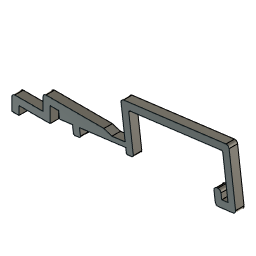
Hook arm over holder v17 (Autodesk Fusion 360 design; units mm, degrees)
Autodesk Fusion 360 part; units mm, degrees
note: some values were not read from the file. Set by a fixed rule: which sketch regions a step uses.
ref_plane "WorkPlane1" through (112.1576, 66, 17) normal (0, 1, 0) x (-1, 0, 0)
sketch "Sketch2" plane through (0, 66, 0) normal (0, 1, 0) x (1, 0, 0)
  line L0 (87, -6) -> (87, -28)
  line L1 (87, -28) -> (130, -28)
  line L2 (130, -28) -> (136, -26)
  line L3 (136, -26) -> (137, -23)
  line L4 (137, -23) -> (98, -18)
  line L5 (98, -18) -> (98, -23)
  line L6 (98, -23) -> (92, -23)
  line L7 (92, -23) -> (92, -6)
  line L8 (92, -6) -> (87, -6)
  constraint vertical L0
  constraint perpendicular L0 L1
  constraint perpendicular L1 L5
  constraint perpendicular L5 L6
  constraint perpendicular L6 L7
  constraint perpendicular L7 L8
extrude "Extrude1" add sketch "Sketch2" along normal blind 6 makes body 1
sketch "Sketch3" plane through (-0.6856, 0, 5.348) normal (0.127164, 0, -0.991882) x (0, 1, 0)
  line L0 (66, 138.8126) -> (66, 99.4934)
  line L1 (66, 99.4934) -> (72, 99.4934)
  line L2 (72, 99.4934) -> (72, 138.8126)
  line L3 (72, 138.8126) -> (66, 138.8126)
  line L4 (69.556, 99.4934) -> (69.556, 104.3824) construction
  line L5 (72, 104.3824) -> (66, 104.3824)
  line L6 (66, 104.3824) -> (66, 109.3824)
  line L7 (66, 109.3824) -> (72, 109.3824)
  line L8 (72, 109.3824) -> (72, 104.3824)
  line L9 (72, 109.3824) -> (66, 109.3824)
  line L10 (66, 109.3824) -> (66, 114.3824)
  line L11 (66, 114.3824) -> (72, 114.3824)
  line L12 (72, 114.3824) -> (72, 109.3824)
  dimension "d4" = 4.889
  dimension "d5" = 5
  dimension "d46" = 5
  constraint coincident L1 L4.start
  constraint perpendicular L1 L4
  constraint horizontal L5
  constraint vertical L6
  constraint horizontal L7
  constraint vertical L8
  constraint coincident L2 L5.start
  constraint horizontal L9
  constraint vertical L10
  constraint horizontal L11
  constraint vertical L12
  constraint coincident L0 L10.end
  measures "d4" distance of L4.start L4.end
  measures "d5" distance of L5.start L7.end
  measures "d46" distance of L7.end L11.end
sketch "Sketch4" plane through (0, 72, 0) normal (0, 1, 0) x (-1, 0, 0)
  line L0 (-137, 23) -> (-98, 18)
  line L1 (-98, 18) -> (-98, 23)
  line L2 (-98, 23) -> (-92, 23)
  line L3 (-92, 23) -> (-92, 6)
  line L4 (-92, 6) -> (-87, 6)
  line L5 (-87, 6) -> (-87, 28)
  line L6 (-87, 28) -> (-130, 28)
  line L7 (-130, 28) -> (-136, 26)
  line L8 (-136, 26) -> (-137, 23)
  line L9 (-87, 6) -> (-92, 6)
  line L10 (-92, 6) -> (-92, 12)
  line L11 (-92, 12) -> (-87, 12)
  line L12 (-87, 12) -> (-87, 6)
  line L13 (-87, 12) -> (-65, 12)
  line L14 (-65, 6) -> (-65, 12)
  line L15 (-65, 17) -> (-87, 17)
  line L16 (-65, 6) -> (-70, 6)
  line L17 (-70, 6) -> (-70, 12)
  line L18 (-70, 12) -> (-65, 12)
  line L19 (-65, 12) -> (-65, 6)
  line L20 (-65, 12) -> (-65, 17)
  constraint horizontal L9
  constraint vertical L10
  constraint horizontal L11
  constraint vertical L12
  constraint coincident L3 L10.end
  constraint coincident L4.end L5.start
  constraint perpendicular L5 L13
  constraint perpendicular L13 L14
  constraint midpoint L5 L15.end
  constraint perpendicular L5 L15
  constraint horizontal L16
  constraint vertical L17
  constraint horizontal L18
  constraint vertical L19
  constraint coincident L13 L17.end
  constraint perpendicular L18 L20
extrude "Extrude3" cut sketch "Sketch4" against normal blind 6.5 contours L3 L4 L5 L9 L10 L11 L12 bodies 1
extrude "Extrude4" add sketch "Sketch4" against normal blind 6 contours L5 L13 L15 L18 L20 | L13 L14 L16 L17 L18 L19 bodies 1
sketch "Sketch5" plane through (-0.6856, 0, 5.348) normal (0.127164, 0, -0.991882) x (0, 1, 0)
  line L0 (72, 99.4934) -> (72, 138.8126)
  line L1 (72, 138.8126) -> (66, 138.8126)
  line L2 (66, 138.8126) -> (66, 99.4934)
  line L3 (69, 109.3824) -> (69, 147.2714) construction
  line L4 (69, 147.2714) -> (66, 147.2714) construction
  line L5 (66, 147.2714) -> (66, 144.7714) construction
  line L6 (66, 144.7714) -> (69, 144.7714) construction
  line L7 (69, 144.7714) -> (69, 147.2714) construction
  line L8 (66, 144.7714) -> (72, 144.7714)
  line L9 (72, 144.7714) -> (72, 149.7714)
  line L10 (72, 149.7714) -> (66, 149.7714)
  line L11 (66, 149.7714) -> (66, 144.7714)
  line L12 (66, 99.4934) -> (72, 99.4934)
  dimension "d21" = 37.889
  dimension "d22" = 2.5
  dimension "d23" = 5
  constraint perpendicular L1 L3
  constraint horizontal L4
  constraint vertical L5
  constraint horizontal L6
  constraint vertical L7
  constraint horizontal L8
  constraint vertical L9
  constraint horizontal L10
  constraint vertical L11
  measures "d21" distance of L3.start L3.end
  measures "d22" distance of L3.end L6.end
  measures "d23" distance of L5.end L10.end
sketch "Sketch6" plane through (0, 66, 0) normal (0, -1, 0) x (1, 0, 0)
  line L0 (65, 17) -> (65, 6)
  line L1 (70, 12) -> (92, 12)
  line L2 (92, 12) -> (92, 23)
  line L3 (92, 23) -> (98, 23)
  line L4 (98, 23) -> (98, 18)
  line L5 (98, 18) -> (137, 23)
  line L6 (137, 23) -> (136, 26)
  line L7 (136, 26) -> (130, 28)
  line L8 (130, 28) -> (87, 28)
  line L9 (87, 28) -> (87, 17)
  line L10 (87, 17) -> (65, 17)
  line L11 (136.0676, 22.8805) -> (135.6529, 26.1157)
  line L12 (65, 6) -> (70, 6)
  line L13 (70, 6) -> (70, 12)
  constraint coincident L5 L11.start
  constraint coincident L7 L11.end
  constraint perpendicular L5 L11
extrude "Extrude5" cut sketch "Sketch6" against normal blind 6.8 contours L5 L6 L7 L11 bodies 1
extrude "Extrude6" add 1 faces at (135.9294, 68, 23.9589) along direction (0.991882, 0, 0.127164) blind 14.461 on bodies 1 bodies 1
sketch "Sketch7" plane through (-1.1004, 0, 8.5832) normal (-0.127164, 0, 0.991882) x (0, -1, 0)
  line L0 (-72, 137.8726) -> (-66, 137.8726)
  line L1 (-66, 137.8726) -> (-66, 152.3336)
  line L2 (-66, 152.3336) -> (-72, 152.3336)
  line L3 (-72, 152.3336) -> (-72, 137.8726)
  line L4 (-66, 152.3336) -> (-72.8279, 152.3336)
  line L5 (-72.8279, 152.3336) -> (-72.8279, 147.3336)
  line L6 (-72.8279, 147.3336) -> (-66, 147.3336)
  line L7 (-66, 147.3336) -> (-66, 152.3336)
  dimension "d30" = 5
  constraint horizontal L4
  constraint vertical L5
  constraint horizontal L6
  constraint vertical L7
  constraint coincident L1.end L2.start
  measures "d30" distance of L1.end L6.end
extrude "Extrude8" add sketch "Sketch7" along normal blind 30 contours L1 L2 L3 L4 L6 L7 bodies 1
sketch "Sketch8" plane through (151.0969, 0, 19.3714) normal (0.991882, 0, 0.127164) x (0, 1, 0)
  line L0 (72, 5.3918) -> (72, 38.6535)
  line L1 (72, 38.6535) -> (66, 38.6535)
  line L2 (66, 38.6535) -> (66, 5.3918)
  line L3 (66, 38.6535) -> (72, 38.6535)
  line L4 (72, 38.6535) -> (72, 33.6535)
  line L5 (72, 33.6535) -> (66, 33.6535)
  line L6 (66, 33.6535) -> (66, 38.6535)
  line L7 (66, 5.3918) -> (72, 5.3918)
  dimension "d33" = 5
  constraint horizontal L3
  constraint vertical L4
  constraint horizontal L5
  constraint vertical L6
  constraint coincident L1.end L2.start
  measures "d33" distance of L1.end L5.end
extrude "Extrude9" add sketch "Sketch8" along normal blind 72 contours L0 L1 L2 L3 L4 L5 L6 bodies 1
sketch "Sketch9" plane through (-4.2795, 0, 33.3803) normal (0.127164, 0, -0.991882) x (0, 1, 0)
  line L0 (66, 152.3336) -> (72, 152.3336)
  line L1 (72, 152.3336) -> (72, 224.3336)
  line L2 (72, 224.3336) -> (66, 224.3336)
  line L3 (66, 224.3336) -> (66, 152.3336)
  line L4 (72, 224.3336) -> (66, 224.3336)
  line L5 (66, 224.3336) -> (66, 219.3336)
  line L6 (66, 219.3336) -> (72, 219.3336)
  line L7 (72, 219.3336) -> (72, 224.3336)
  dimension "d36" = 5
  constraint horizontal L4
  constraint vertical L5
  constraint horizontal L6
  constraint vertical L7
  constraint coincident L3 L5.end
  constraint coincident L1.end L2.start
  measures "d36" distance of L1.end L6.end
extrude "Extrude10" add sketch "Sketch9" along normal blind 40 contours L1 L2 L3 L4 L5 L6 L7 bodies 1
sketch "Sketch10" plane through (0.807, 0, -6.295) normal (0.127164, 0, -0.991882) x (0, 1, 0)
  line L0 (72, 219.3336) -> (72, 224.3336)
  line L1 (72, 224.3336) -> (66, 224.3336)
  line L2 (66, 224.3336) -> (66, 219.3336)
  line L3 (66, 219.3336) -> (72, 219.3336)
  line L4 (66, 219.3336) -> (72.721, 219.3336)
  line L5 (66, 214.8336) -> (66, 219.3336)
  line L6 (72, 219.3336) -> (66, 219.3336)
  line L7 (66, 219.3336) -> (66, 214.8336)
  line L8 (66, 214.8336) -> (72, 214.8336)
  line L9 (72, 214.8336) -> (72, 219.3336)
  line L10 (66, 214.8336) -> (72, 214.8336)
  line L11 (72, 214.8336) -> (72, 209.8336)
  line L12 (72, 209.8336) -> (66, 209.8336)
  line L13 (66, 209.8336) -> (66, 214.8336)
  dimension "d40" = 6
  dimension "d41" = 4.5
  dimension "d56" = 5
  constraint horizontal L4
  constraint vertical L5
  constraint coincident L2.end L3.start
  constraint horizontal L6
  constraint vertical L7
  constraint horizontal L8
  constraint vertical L9
  constraint coincident L0.start L3.end
  constraint horizontal L10
  constraint vertical L11
  constraint horizontal L12
  constraint vertical L13
  measures "d40" distance of L0.start L2.end
  measures "d41" distance of L0.start L8.end
  measures "d56" distance of L5.start L12.end
extrude "Extrude11" add sketch "Sketch10" against normal blind 5 contours L3 L4 L5 L6 L7 L8 L9 L10 bodies 1
extrude "Extrude13" add sketch "Sketch3" along normal blind 6 contours L0 L2 L7 L9 L10 L11 L12 bodies 1
sketch "Sketch11" plane through (-0.6856, 0, 5.348) normal (0.127164, 0, -0.991882) x (0, 1, 0)
  line L0 (66, 114.3824) -> (72, 114.3824)
  line L1 (72, 114.3824) -> (72, 152.3336)
  line L2 (72, 152.3336) -> (66, 152.3336)
  line L3 (66, 152.3336) -> (66, 114.3824)
  line L4 (72, 152.3336) -> (65.9909, 152.3336)
  line L5 (65.9909, 152.3336) -> (65.9909, 147.3336)
  line L6 (65.9909, 147.3336) -> (72, 147.3336)
  line L7 (72, 147.3336) -> (72, 152.3336)
  dimension "d49" = 5
  constraint horizontal L4
  constraint vertical L5
  constraint horizontal L6
  constraint vertical L7
  constraint coincident L1.end L2.start
  measures "d49" distance of L1.end L6.end
extrude "Extrude14" add sketch "Sketch11" along normal blind 4 contours L1 L2 L3 L4 L6 L7 bodies 1
fillet "Fillet4" radius 1 2 edges at (113.5311, 69, 13.9421) (108.5717, 69, 13.3062) on bodies 1
fillet "Fillet5" radius 1 2 edges at (145.9605, 69, 20.116) (150.9199, 69, 20.7519) on bodies 1
extrude "Extrude15" add sketch "Sketch10" against normal blind 11 separate body contours L8 L10 L11 L12 L13 makes body 2
fillet "Fillet6" radius 2 4 edges at (223.3194, 69, 22.2322) (212.4977, 69, 31.9349) (207.5383, 69, 31.2991) (208.9371, 69, 20.3884) on bodies 1 2
sketch "Sketch12" plane through (0, 66, 0) normal (0, -1, 0) x (1, 0, 0)
  arc A0 (221.3356, 21.9779) -> (223.0651, 24.216) centre (221.0813, 23.9617) ccw
  line L0 (223.0651, 24.216) -> (217.597, 66.8669)
  line L1 (217.597, 66.8669) -> (141.2221, 57.0753)
  line L2 (141.2221, 57.0753) -> (145.037, 27.3188)
  line L3 (145.037, 27.3188) -> (135.6529, 26.1157)
  line L4 (135.6529, 26.1157) -> (130, 28)
  line L5 (130, 28) -> (87, 28)
  line L6 (87, 28) -> (87, 17)
  line L7 (87, 17) -> (65, 17)
  line L8 (65, 17) -> (65, 6)
  line L9 (65, 6) -> (70, 6)
  line L10 (70, 6) -> (70, 12)
  line L11 (70, 12) -> (92, 12)
  line L12 (92, 12) -> (92, 23)
  line L13 (92, 23) -> (98, 23)
  line L14 (98, 23) -> (98, 18)
  line L15 (98, 18) -> (107.8087, 19.2575)
  line L16 (107.8087, 19.2575) -> (108.4445, 14.2981)
  arc A1 (108.4445, 14.2981) -> (109.5636, 13.4334) centre (109.4364, 14.4253) ccw
  line L17 (109.5636, 13.4334) -> (112.5392, 13.8149)
  arc A2 (112.5392, 13.8149) -> (113.4039, 14.9339) centre (112.4121, 14.8068) ccw
  line L18 (113.4039, 14.9339) -> (112.7681, 19.8933)
  line L19 (112.7681, 19.8933) -> (145.4518, 24.0836)
  line L20 (145.4518, 24.0836) -> (145.8333, 21.1079)
  arc A3 (145.8333, 21.1079) -> (146.9524, 20.2432) centre (146.8252, 21.2351) ccw
  line L21 (146.9524, 20.2432) -> (149.928, 20.6247)
  arc A4 (149.928, 20.6247) -> (150.7927, 21.7437) centre (149.8008, 21.6166) ccw
  line L22 (150.7927, 21.7437) -> (146.8173, 52.7517)
  line L23 (146.8173, 52.7517) -> (213.2734, 61.2717)
  line L24 (213.2734, 61.2717) -> (217.7242, 26.5558)
  line L25 (217.7242, 26.5558) -> (213.2607, 25.9836)
  line L26 (213.2607, 25.9836) -> (213.8965, 21.0242)
  line L27 (213.8965, 21.0242) -> (221.3356, 21.9779)
  line L28 (98, 23) -> (98.6307, 18.0809)
  constraint coincident L13.end L14.start
  constraint coincident L15 L28.end
  constraint perpendicular L15 L28
extrude "Extrude16" cut sketch "Sketch12" against normal blind 8 contours L14 L15 L28 bodies 1
fillet "Fillet7" radius 2 2 edges at (87, 69, 28) (65, 69, 17) on bodies 1
fillet "Fillet8" radius 2 2 edges at (141.2221, 69, 57.0753) (217.597, 69, 66.8669) on bodies 1
fillet "Fillet8" radius 2.5 2 edges at (146.8173, 69, 52.7517) (213.2734, 69, 61.2717) on bodies 1
sketch "Sketch13" plane through (0, 66, 0) normal (0, -1, 0) x (1, 0, 0)
  arc A0 (217.8513, 64.8832) -> (215.6132, 66.6126) centre (215.8676, 64.6288) ccw
  line L0 (215.6132, 66.6126) -> (143.2059, 57.3296)
  arc A1 (143.2059, 57.3296) -> (141.4764, 55.0915) centre (143.4602, 55.3458) ccw
  line L1 (141.4764, 55.0915) -> (145.037, 27.3188)
  line L2 (145.037, 27.3188) -> (135.6529, 26.1157)
  line L3 (135.6529, 26.1157) -> (130, 28)
  line L4 (130, 28) -> (89, 28)
  arc A2 (89, 28) -> (87, 26) centre (89, 26) ccw
  line L5 (87, 26) -> (87, 17)
  line L6 (87, 17) -> (67, 17)
  arc A3 (67, 17) -> (65, 15) centre (67, 15) ccw
  line L7 (65, 15) -> (65, 6)
  line L8 (65, 6) -> (70, 6)
  line L9 (70, 6) -> (70, 12)
  line L10 (70, 12) -> (92, 12)
  line L11 (92, 12) -> (92, 23)
  line L12 (92, 23) -> (98, 23)
  line L13 (98, 23) -> (98.6307, 18.0809)
  line L14 (98.6307, 18.0809) -> (107.8087, 19.2575)
  line L15 (107.8087, 19.2575) -> (108.4445, 14.2981)
  arc A4 (108.4445, 14.2981) -> (109.5636, 13.4334) centre (109.4364, 14.4253) ccw
  line L16 (109.5636, 13.4334) -> (112.5392, 13.8149)
  arc A5 (112.5392, 13.8149) -> (113.4039, 14.9339) centre (112.4121, 14.8068) ccw
  line L17 (113.4039, 14.9339) -> (112.7681, 19.8933)
  line L18 (112.7681, 19.8933) -> (145.4518, 24.0836)
  line L19 (145.4518, 24.0836) -> (145.8333, 21.1079)
  arc A6 (145.8333, 21.1079) -> (146.9524, 20.2432) centre (146.8252, 21.2351) ccw
  line L20 (146.9524, 20.2432) -> (149.928, 20.6247)
  arc A7 (149.928, 20.6247) -> (150.7927, 21.7437) centre (149.8008, 21.6166) ccw
  line L21 (150.7927, 21.7437) -> (147.1353, 50.272)
  arc A8 (149.2971, 53.0696) -> (147.1353, 50.272) centre (149.615, 50.5899) ccw
  line L22 (149.2971, 53.0696) -> (210.7937, 60.9538)
  arc A9 (213.5913, 58.792) -> (210.7937, 60.9538) centre (211.1116, 58.4741) ccw
  line L23 (213.5913, 58.792) -> (217.7242, 26.5558)
  line L24 (217.7242, 26.5558) -> (213.2607, 25.9836)
  line L25 (213.2607, 25.9836) -> (213.8965, 21.0242)
  line L26 (213.8965, 21.0242) -> (221.3356, 21.9779)
  arc A10 (221.3356, 21.9779) -> (223.0651, 24.216) centre (221.0813, 23.9617) ccw
  line L27 (223.0651, 24.216) -> (217.8513, 64.8832)
  line L28 (180.0454, 57.0117) -> (180.6812, 52.0523)
  line L29 (180.6812, 52.0523) -> (213.9092, 56.3123)
  line L30 (180.6812, 52.0523) -> (147.4532, 47.7923)
  dimension "d69" = 5
  constraint midpoint L22 L28.start
  constraint perpendicular L22 L28
  constraint coincident L23 L29.end
  constraint perpendicular L23 L29
  constraint coincident L21 L30.end
  constraint perpendicular L21 L30
  measures "d69" distance of L28.start L28.end
extrude "Extrude17" add sketch "Sketch13" against normal blind 6 contours L22 A9 L23 L28 L29 | L21 A8 L22 L28 L30 bodies 1
sketch "Sketch14" plane through (0, 66, 0) normal (0, -1, 0) x (1, 0, 0)
  arc A0 (217.8513, 64.8832) -> (215.6132, 66.6126) centre (215.8676, 64.6288) ccw
  line L0 (215.6132, 66.6126) -> (143.2059, 57.3296)
  arc A1 (143.2059, 57.3296) -> (141.4764, 55.0915) centre (143.4602, 55.3458) ccw
  line L1 (141.4764, 55.0915) -> (145.037, 27.3188)
  line L2 (145.037, 27.3188) -> (135.6529, 26.1157)
  line L3 (135.6529, 26.1157) -> (130, 28)
  line L4 (130, 28) -> (89, 28)
  arc A2 (89, 28) -> (87, 26) centre (89, 26) ccw
  line L5 (87, 26) -> (87, 17)
  line L6 (87, 17) -> (67, 17)
  arc A3 (67, 17) -> (65, 15) centre (67, 15) ccw
  line L7 (65, 15) -> (65, 6)
  line L8 (65, 6) -> (70, 6)
  line L9 (70, 6) -> (70, 12)
  line L10 (70, 12) -> (92, 12)
  line L11 (92, 12) -> (92, 23)
  line L12 (92, 23) -> (98, 23)
  line L13 (98, 23) -> (98.6307, 18.0809)
  line L14 (98.6307, 18.0809) -> (107.8087, 19.2575)
  line L15 (107.8087, 19.2575) -> (108.4445, 14.2981)
  arc A4 (108.4445, 14.2981) -> (109.5636, 13.4334) centre (109.4364, 14.4253) ccw
  line L16 (109.5636, 13.4334) -> (112.5392, 13.8149)
  arc A5 (112.5392, 13.8149) -> (113.4039, 14.9339) centre (112.4121, 14.8068) ccw
  line L17 (113.4039, 14.9339) -> (112.7681, 19.8933)
  line L18 (112.7681, 19.8933) -> (145.4518, 24.0836)
  line L19 (145.4518, 24.0836) -> (145.8333, 21.1079)
  arc A6 (145.8333, 21.1079) -> (146.9524, 20.2432) centre (146.8252, 21.2351) ccw
  line L20 (146.9524, 20.2432) -> (149.928, 20.6247)
  arc A7 (149.928, 20.6247) -> (150.7927, 21.7437) centre (149.8008, 21.6166) ccw
  line L21 (150.7927, 21.7437) -> (147.4532, 47.7923)
  line L22 (147.4532, 47.7923) -> (213.9092, 56.3123)
  line L23 (213.9092, 56.3123) -> (217.7242, 26.5558)
  line L24 (217.7242, 26.5558) -> (213.2607, 25.9836)
  line L25 (213.2607, 25.9836) -> (213.8965, 21.0242)
  line L26 (213.8965, 21.0242) -> (221.3356, 21.9779)
  arc A8 (221.3356, 21.9779) -> (223.0651, 24.216) centre (221.0813, 23.9617) ccw
  line L27 (223.0651, 24.216) -> (217.8513, 64.8832)
  line L28 (213.9092, 56.3123) -> (213.2734, 61.2717) construction
  line L29 (213.2734, 61.2717) -> (141.8579, 52.1159) construction
  line L30 (141.8579, 52.1159) -> (218.2328, 61.9075)
  dimension "d72" = 5
  constraint coincident L22.end L23.start
  constraint perpendicular L22 L28
  constraint coincident L1 L29.end
  constraint perpendicular L1 L29
  constraint coincident L27 L30.end
  constraint perpendicular L27 L30
  measures "d72" distance of L22.end L28.end
extrude "Extrude18" cut sketch "Sketch14" against normal blind 10 contours A0 L0 A1 L1 L27 L30 bodies 1
fillet "Fillet9" radius 2 2 edges at (218.2328, 69, 61.9075) (141.8579, 69, 52.1159) on bodies 1
fillet "Fillet10" radius 1 2 edges at (213.9092, 69, 56.3123) (147.4532, 69, 47.7923) on bodies 1
combine "Combine1" operation add target body 2 tool bodies 1
sketch "Sketch15" plane through (0, 66, 0) normal (0, -1, 0) x (1, 0, 0)
  arc A0 (208.6828, 22.3721) -> (210.9209, 20.6427) centre (210.6666, 22.6265) ccw
  line L0 (210.9209, 20.6427) -> (221.3356, 21.9779)
  arc A1 (221.3356, 21.9779) -> (223.0651, 24.216) centre (221.0813, 23.9617) ccw
  line L1 (223.0651, 24.216) -> (218.4872, 59.9237)
  arc A2 (218.4872, 59.9237) -> (216.2491, 61.6532) centre (216.5034, 59.6694) ccw
  line L2 (216.2491, 61.6532) -> (143.8417, 52.3702)
  arc A3 (143.8417, 52.3702) -> (142.1123, 50.1321) centre (144.096, 50.3864) ccw
  line L3 (142.1123, 50.1321) -> (145.037, 27.3188)
  line L4 (145.037, 27.3188) -> (135.6529, 26.1157)
  line L5 (135.6529, 26.1157) -> (130, 28)
  line L6 (130, 28) -> (89, 28)
  arc A4 (89, 28) -> (87, 26) centre (89, 26) ccw
  line L7 (87, 26) -> (87, 17)
  line L8 (87, 17) -> (67, 17)
  arc A5 (67, 17) -> (65, 15) centre (67, 15) ccw
  line L9 (65, 15) -> (65, 6)
  line L10 (65, 6) -> (70, 6)
  line L11 (70, 6) -> (70, 12)
  line L12 (70, 12) -> (92, 12)
  line L13 (92, 12) -> (92, 23)
  line L14 (92, 23) -> (98, 23)
  line L15 (98, 23) -> (98.6307, 18.0809)
  line L16 (98.6307, 18.0809) -> (107.8087, 19.2575)
  line L17 (107.8087, 19.2575) -> (108.4445, 14.2981)
  arc A6 (108.4445, 14.2981) -> (109.5636, 13.4334) centre (109.4364, 14.4253) ccw
  line L18 (109.5636, 13.4334) -> (112.5392, 13.8149)
  arc A7 (112.5392, 13.8149) -> (113.4039, 14.9339) centre (112.4121, 14.8068) ccw
  line L19 (113.4039, 14.9339) -> (112.7681, 19.8933)
  line L20 (112.7681, 19.8933) -> (145.4518, 24.0836)
  line L21 (145.4518, 24.0836) -> (145.8333, 21.1079)
  arc A8 (145.8333, 21.1079) -> (146.9524, 20.2432) centre (146.8252, 21.2351) ccw
  line L22 (146.9524, 20.2432) -> (149.928, 20.6247)
  arc A9 (149.928, 20.6247) -> (150.7927, 21.7437) centre (149.8008, 21.6166) ccw
  line L23 (150.7927, 21.7437) -> (147.5803, 46.8004)
  arc A10 (148.4451, 47.9194) -> (147.5803, 46.8004) centre (148.5722, 46.9276) ccw
  line L24 (148.4451, 47.9194) -> (212.9174, 56.1851)
  arc A11 (214.0364, 55.3204) -> (212.9174, 56.1851) centre (213.0445, 55.1932) ccw
  line L25 (214.0364, 55.3204) -> (217.7242, 26.5558)
  line L26 (217.7242, 26.5558) -> (213.2607, 25.9836)
  line L27 (213.2607, 25.9836) -> (212.752, 29.9511)
  arc A12 (212.752, 29.9511) -> (210.514, 31.6806) centre (210.7683, 29.6968) ccw
  line L28 (210.514, 31.6806) -> (209.5221, 31.5534)
  arc A13 (209.5221, 31.5534) -> (207.7926, 29.3153) centre (209.7764, 29.5696) ccw
  line L29 (207.7926, 29.3153) -> (208.6828, 22.3721)
